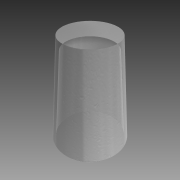
# Autodesk Inventor part: CocktailGlas
Saved by Autodesk Inventor 2013 (Build 170138000, 138)
## iProperties
Created: 2012-10-19
Part Number: CocktailGlas
Material: Acryl, farblos
Document SubType Name: Modeling
Designer: fivef
Density: 1.19 g/cm^3
Mass: 148.34 g
Surface Area: 546.855 cm^2
Volume: 124.656 cm^3
Author: fivef
Autodesk Inventor part; units mm, degrees
ref_plane "YZ Plane" through (0, 0, 0) normal (1, 0, 0) x (0, 1, 0)
ref_plane "XZ Plane" through (0, 0, 0) normal (0, 1, 0) x (-1, 0, 0)
ref_plane "XY Plane" through (0, 0, 0) normal (0, 0, 1) x (1, 0, 0)
sketch "Skizze2" plane through (0, 0, 0) normal (0, 1, 0) x (-1, 0, 0)
  line L0 (0, 0) -> (-30, 0)
  line L1 (0, 0) -> (0, -120) construction
  line L2 (-41.5, -120) -> (0, -120) construction
  line L3 (-30, 0) -> (-41.3163, -118.0831)
  line L4 (0, -15) -> (0, 0)
  line L5 (0, -15) -> (-27.9215, -15)
  line L6 (-27.9215, -15) -> (-37.8323, -118.4169)
  arc A0 (-41.3163, -118.0831) -> (-37.8323, -118.4169) centre (-39.5743, -118.25) ccw
  dimension "d0" = 30
  dimension "d4" = 120
  dimension "d5" = 41.5
  dimension "d6" = 15
  dimension "d7" = 3.5
  constraints: 14 end point, 3 tangent, 2 parallel, 2 perpendicular, 2 point on circle, 1 centre point, 1 coincident, 1 point on line
  measures "d0" distance of L0.start L0.end
  measures "d4" distance of L0.start L1.end
  measures "d5" distance of L1.end L2.start
  measures "d6" distance of L0.start L4.start
  measures "d7" distance between parallel lines of L6 L3
revolve "Umdrehung1" add sketch "Skizze2" angle 360 about axis through (0, 0, 0) along (0, 0, -1)
